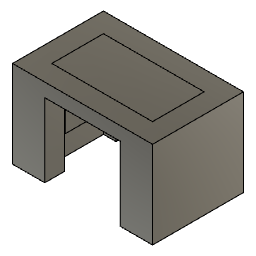
Servo housing (Autodesk Fusion 360 design; units mm, degrees)
Autodesk Fusion 360 part; units mm, degrees
sketch "Sketch1" plane through (0, 0, 0) normal (0, 0, 1) x (1, 0, 0)
  line L0 (0, 0) -> (57, 0)
  line L1 (57, 0) -> (57, -37)
  line L2 (57, -37) -> (0, -37)
  line L3 (0, -37) -> (0, 0)
  line L4 (8, -8) -> (49, -8)
  line L5 (49, -8) -> (49, -29)
  line L6 (49, -29) -> (8, -29)
  line L7 (8, -29) -> (8, -8)
  dimension "d7" = 57
  dimension "d8" = 37
  dimension "d15" = 21
  dimension "d16" = 41
  dimension "d17" = 8
  dimension "d18" = 8
  constraint horizontal L0
  constraint vertical L1
  constraint horizontal L2
  constraint vertical L3
  constraint coincident L0.start L3.end
  constraint horizontal L4
  constraint vertical L5
  constraint horizontal L6
  constraint vertical L7
  measures "d7" distance of L0.start L0.end
  measures "d8" distance of L0.start L2.end
  measures "d15" distance of L4.start L6.end
  measures "d16" distance of L4.start L4.end
  measures "d17" distance of L0 L4
  measures "d18" distance of L3 L7
extrude "Extrude2" add sketch "Sketch1" along normal blind 35.5 makes body 1
extrude "Extrude1" add sketch "Sketch1" along normal blind 35.5 separate body contours L0 L1 L2 L3 | L4 L5 L6 L7 makes body 2
extrude "Extrude3" cut sketch "Sketch1" along normal blind 30 contours L4 L5 L6 L7 bodies 2
sketch "Sketch3" plane through (0, -37, 0) normal (0, -1, 0) x (1, 0, 0)
  line L0 (0, 0) -> (57, 0)
  line L1 (57, 0) -> (57, 35.5)
  line L2 (57, 35.5) -> (0, 35.5)
  line L3 (0, 35.5) -> (0, 0)
  line L4 (13.125, 30) -> (43.875, 30)
  line L5 (43.875, 30) -> (43.875, -5.5)
  line L6 (43.875, -5.5) -> (13.125, -5.5)
  line L7 (13.125, -5.5) -> (13.125, 30)
  dimension "d26" = 30.75
  dimension "d27" = 35.5
  dimension "d28" = 5.5
  dimension "d32" = 13.125
  constraint horizontal L4
  constraint vertical L5
  constraint horizontal L6
  constraint vertical L7
  measures "d26" distance of L4.start L4.end
  measures "d27" distance of L4.start L6.end
  measures "d28" distance of L2 L4
  measures "d32" distance of L1 L5
extrude "Extrude4" cut sketch "Sketch3" against normal blind 100 contours L0 L4 L5 L7 | L0 L5 L6 L7 bodies 1 2
sketch "Sketch4" plane through (0, 0, 0) normal (-1, 0, 0) x (0, -1, 0)
  line L0 (0, 0) -> (37, 0)
  line L1 (37, 0) -> (37, 35.5)
  line L2 (37, 35.5) -> (0, 35.5)
  line L3 (0, 35.5) -> (0, 0)
  line L4 (13.5, 30) -> (23.5, 30)
  line L5 (23.5, 30) -> (23.5, 8)
  line L6 (23.5, 8) -> (13.5, 8)
  line L7 (13.5, 8) -> (13.5, 30)
  line L8 (37, 0) -> (0, 0)
  line L9 (37, -5.5) -> (37, 30)
  dimension "d36" = 10
  dimension "d37" = 22
  dimension "d40" = 13.5
  dimension "d43" = 5.5
  constraint horizontal L4
  constraint vertical L5
  constraint horizontal L6
  constraint vertical L7
  measures "d36" distance of L4.start L4.end
  measures "d37" distance of L4.start L6.end
  measures "d40" distance of L5 L9
  measures "d43" distance of L2 L4
extrude "Extrude5" cut sketch "Sketch4" against normal blind 13 contours L4 L5 L6 L7 bodies 1 2
equation "bottom_thickness = 5.5 mm"
equation "side_thickness = 8 mm"
equation "outer_width = 37 mm"
equation "height = 30 mm + bottom_thickness"
equation "outer_length = 57 mm"
equation "inner_length = outer_length - 2 * side_thickness"
equation "d7 = outer_length"
equation "d8 = outer_width"
equation "d9 = height"
equation "inner_width = outer_width - 2 * side_thickness"
equation "d15 = inner_width"
equation "d16 = inner_length"
equation "d17 = side_thickness"
equation "d18 = side_thickness"
equation "d19 = height"
equation "d21 = height - bottom_thickness"
equation "big_side_gap = 3 * inner_length / 4"
equation "big_side_gap_distance = ( outer_length - big_side_gap ) / 2"
equation "extra = 100 mm"
equation "d26 = big_side_gap"
equation "d27 = height"
equation "d28 = bottom_thickness"
equation "d30 = -extra"
equation "d32 = big_side_gap_distance"
equation "small_side_gap_width = 22 mm"
equation "small_side_gap_length = 10 mm"
equation "small_side_gap_depth = side_thickness + 5 mm"
equation "d36 = small_side_gap_length"
equation "d37 = small_side_gap_width"
equation "small_side_gap_distance = ( outer_width - small_side_gap_length ) / 2"
equation "d40 = small_side_gap_distance"
equation "d41 = -small_side_gap_depth"
equation "d43 = bottom_thickness"
equation "cable_dent = 5 mm"
